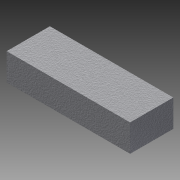
# Autodesk Inventor part: Battery
Saved by Autodesk Inventor 2015 (Build 190159000, 159)
## iProperties
Created: 2015-05-24
Part Number: Battery
Material: コンクリート
Document SubType Name: Modeling
Designer: kenta
Density: 1.97874 g/cm^3
Appearance: 露出材 砂利 - 粗い
Mass: 152.363 g
Surface Area: 129.4 cm^2
Volume: 77 cm^3
Author: kenta
Autodesk Inventor part; units mm, degrees
ref_plane "YZ Plane" through (0, 0, 0) normal (1, 0, 0) x (0, 1, 0)
ref_plane "XZ Plane" through (0, 0, 0) normal (0, 1, 0) x (-1, 0, 0)
ref_plane "XY Plane" through (0, 0, 0) normal (0, 0, 1) x (1, 0, 0)
sketch "スケッチ1" plane through (0, 0, 0) normal (0, 0, 1) x (1, 0, 0)
  line L0 (-50, 17.5) -> (50, 17.5)
  line L1 (50, 17.5) -> (50, -17.5)
  line L2 (50, -17.5) -> (-50, -17.5)
  line L3 (-50, -17.5) -> (-50, 17.5)
  line L4 (-50, 17.5) -> (50, -17.5) construction
  line L5 (50, 17.5) -> (-50, -17.5) construction
  point P0 (0, 0)
  dimension "d0" = 100
  dimension "d1" = 35
  constraints: 12 end point, 2 midpoint, 2 parallel, 1 horizontal, 1 perpendicular
  measures "d0" distance of L1.end L2.end
  measures "d1" distance of L0.end L1.end
extrude "押し出し1" add sketch "スケッチ1" along normal blind 22
